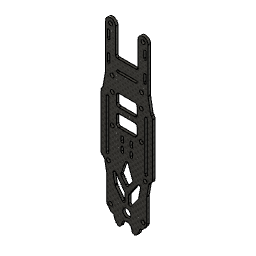
VTX_Mount_Assembly (Autodesk Fusion 360 archive; units mm, degrees)
design "frame_top_2mm"
Autodesk Fusion 360 part; units mm, degrees
(part 1 of 3)
sketch "Sketch1" plane through (0, 0, 0) normal (0, 0, 1) x (1, 0, 0)
  circle A0 centre (15.25, -31.25) radius 1.6
  line L0 (2, 0) -> (13.2991, 0) construction
  line L1 (2, 0) -> (13.2991, 0) construction
  line L2 (9.35, 67.3) -> (9.35, 67.95)
  line L3 (15.95, 56.45) -> (15.95, 62.15)
  circle A1 centre (13.5, 67.95) radius 1.6
  circle A2 centre (13.5, 67.95) radius 4.15
  arc A3 (14.15, 56.45) -> (15.95, 56.45) centre (15.05, 56.45) ccw
  line L4 (14.15, 62.15) -> (14.15, 56.45)
  circle A4 centre (12.2, 31.25) radius 1.6
  line L5 (15.05, 62.15) -> (15.05, 56.45) construction
  arc A5 (15.95, 62.15) -> (14.15, 62.15) centre (15.05, 62.15) ccw
  circle A6 centre (13.45, -61.45) radius 1.6
  line L6 (13.5, 72.1) -> (-2.7063, 72.1) construction
  line L7 (0, 45.6) -> (7.85, 45.6)
  line L8 (9.35, 47.1) -> (9.35, 67.95)
  line L9 (9.35, 67.95) -> (0, 67.95)
  line L10 (0, 67.95) -> (0, 45.6)
  arc A7 (7.85, 45.6) -> (9.35, 47.1) centre (7.85, 47.1) ccw
  circle A8 centre (12, 19.45) radius 1.6
  circle A9 centre (12, -4.55) radius 1.6
  line L11 (17.65, 67.95) -> (17.65, 30.95)
  line L12 (15.95, 39.45) -> (15.95, 45.15)
  arc A10 (15.95, 45.15) -> (14.15, 45.15) centre (15.05, 45.15) ccw
  line L13 (14.15, 45.15) -> (14.15, 39.45)
  line L14 (15.05, 45.15) -> (15.05, 39.45) construction
  arc A11 (14.15, 39.45) -> (15.95, 39.45) centre (15.05, 39.45) ccw
  line L15 (17.65, 30.95) -> (20.0688, 17.2322)
  line L16 (21.35, 19.1304) -> (21.35, -33.1855)
  line L17 (21.35, 17.5398) -> (19.8632, 18.3982)
  circle A12 centre (13.45, -61.45) radius 3.1
  line L18 (16.55, -61.45) -> (16.55, -41.45)
  line L19 (16.55, -41.45) -> (18.6024, -29.8104)
  line L20 (16.55, -41.45) -> (28.3691, -41.45) construction
  line L21 (21.35, -29.1237) -> (18.4258, -30.812)
  line L22 (21.35, -29.1237) -> (17.9734, -29.1237) construction
  arc A13 (11.4643, -67.4123) -> (14.739, -64.2693) centre (10.8143, -63.4576) ccw
  circle A14 centre (0, -71.85) radius 4.25
  line L23 (0, -71.85) -> (0, 0) construction
  line L24 (10.8143, -67.4654) -> (8.5812, -67.4654) construction
  line L25 (6.7155, -73.9955) -> (4.3713, -73.9955) construction
  spline S0 degree 5 poles (10.6535, -68.1682) (10.6286, -68.2734) (10.547, -68.6119) (10.4102, -69.1517) (10.2203, -69.8303) (9.9795, -70.5538) (9.7046, -71.1854) (9.4084, -71.6765) (9.0557, -72.1429) (8.6004, -72.7445) (8.0471, -73.3833) (7.5409, -73.7918) (7.1365, -73.9585) (6.8574, -73.9955) (6.7155, -73.9955) knots 0.056122 0.056122 0.056122 0.056122 0.056122 0.056122 0.1 0.2 0.3 0.4 0.5 0.6 0.7 0.8 0.9 1 1 1 1 1 1
  line L26 (9.6717, -71.2822) -> (8.91, -72.3592)
  arc A15 (4.2449, -71.6427) -> (6.7155, -73.9955) centre (6.7155, -71.5221) ccw
  arc A16 (11.4643, -67.4123) -> (10.6535, -68.1682) centre (11.6265, -68.3991) ccw
  circle A17 centre (0, -61.45) radius 3.35
  line L27 (0, -61.45) -> (13.45, -61.45) construction
  line L28 (-7.55, 35.5) -> (7.55, 35.5)
  arc A18 (7.55, 35.5) -> (7.55, 37.4) centre (7.55, 36.45) ccw
  line L29 (7.55, 37.4) -> (-7.55, 37.4)
  arc A19 (-7.55, 37.4) -> (-7.55, 35.5) centre (-7.55, 36.45) ccw
  line L30 (-8.5, 36.45) -> (8.5, 36.45) construction
  line L31 (0, 36.45) -> (0, 0) construction
  line L32 (-6.6, 21.2) -> (6.6, 21.2)
  line L33 (8.6, 19.2) -> (8.6, 13)
  line L34 (6.6, 11) -> (-6.6, 11)
  line L35 (-8.6, 13) -> (-8.6, 19.2)
  line L36 (-8.6, 21.2) -> (8.6, 11) construction
  line L37 (8.6, 21.2) -> (-8.6, 11) construction
  line L38 (-6.6, 6.6) -> (6.6, 6.6)
  line L39 (8.6, 4.6) -> (8.6, -1.6)
  line L40 (6.6, -3.6) -> (-6.6, -3.6)
  line L41 (-8.6, -1.6) -> (-8.6, 4.6)
  line L42 (-8.6, 6.6) -> (8.6, -3.6) construction
  line L43 (8.6, 6.6) -> (-8.6, -3.6) construction
  arc A20 (-6.6, 6.6) -> (-8.6, 4.6) centre (-6.6, 4.6) ccw
  arc A21 (-8.6, -1.6) -> (-6.6, -3.6) centre (-6.6, -1.6) ccw
  arc A22 (6.6, -3.6) -> (8.6, -1.6) centre (6.6, -1.6) ccw
  arc A23 (8.6, 4.6) -> (6.6, 6.6) centre (6.6, 4.6) ccw
  arc A24 (6.6, 11) -> (8.6, 13) centre (6.6, 13) ccw
  arc A25 (-8.6, 13) -> (-6.6, 11) centre (-6.6, 13) ccw
  arc A26 (-6.6, 21.2) -> (-8.6, 19.2) centre (-6.6, 19.2) ccw
  arc A27 (8.6, 19.2) -> (6.6, 21.2) centre (6.6, 19.2) ccw
  line L44 (2.75, -8.9) -> (2.75, -12)
  arc A28 (2.75, -12) -> (4.75, -12) centre (3.75, -12) ccw
  line L45 (4.75, -12) -> (4.75, -8.9)
  arc A29 (4.75, -8.9) -> (2.75, -8.9) centre (3.75, -8.9) ccw
  line L46 (3.75, -7.9) -> (3.75, -13) construction
  line L47 (2.75, -16.5) -> (2.75, -19.6)
  arc A30 (4.75, -16.5) -> (2.75, -16.5) centre (3.75, -16.5) ccw
  line L48 (3.75, -15.5) -> (3.75, -20.6) construction
  arc A31 (2.75, -19.6) -> (4.75, -19.6) centre (3.75, -19.6) ccw
  line L49 (4.75, -19.6) -> (4.75, -16.5)
  line L50 (14.95, 14.45) -> (14.95, -26.05)
  arc A32 (14.95, -26.05) -> (16.95, -26.05) centre (15.95, -26.05) ccw
  line L51 (16.95, -26.05) -> (16.95, 14.45)
  arc A33 (16.95, 14.45) -> (14.95, 14.45) centre (15.95, 14.45) ccw
  line L52 (15.95, 15.45) -> (15.95, -27.05) construction
  line L53 (0, -22.2) -> (5.1, -36.2121)
  line L54 (5.1, -36.2121) -> (0, -43.2)
  line L55 (1.45, -54.0214) -> (1.45, -48.0614)
  line L56 (1.6739, -47.3475) -> (10.5932, -34.5275)
  line L57 (9.8726, -46.033) -> (12.1558, -33.9583)
  line L58 (9.6573, -46.5332) -> (3.7129, -54.7538)
  arc A34 (11.3939, -37.9877) -> (8.9108, -36.9456) centre (10.041, -37.7319) ccw
  arc A35 (9.6573, -46.5332) -> (9.8726, -46.033) centre (8.6443, -45.8007) ccw
  arc A36 (1.6739, -47.3475) -> (1.45, -48.0614) centre (2.7, -48.0614) ccw
  arc A37 (1.45, -54.0214) -> (3.7129, -54.7538) centre (2.7, -54.0214) ccw
  arc A38 (-8.6, 13) -> (-6.6, 11) centre (-6.6, 13) ccw
  arc A39 (-15.95, 39.45) -> (-14.15, 39.45) centre (-15.05, 39.45) ccw
  line L59 (0, 67.95) -> (0, 45.6)
  line L60 (0, 36.45) -> (0, 0) construction
  circle A40 centre (-13.45, -61.45) radius 1.6
  line L61 (-3.75, -15.5) -> (-3.75, -20.6) construction
  arc A41 (-1.45, -48.0614) -> (-1.6739, -47.3475) centre (-2.7, -48.0614) ccw
  arc A42 (-4.75, -12) -> (-2.75, -12) centre (-3.75, -12) ccw
  line L62 (-21.35, -29.1237) -> (-17.9734, -29.1237) construction
  line L63 (-16.55, -41.45) -> (-18.6024, -29.8104)
  line L64 (-4.75, -19.6) -> (-4.75, -16.5)
  circle A43 centre (-15.25, -31.25) radius 1.6
  line L65 (-14.15, 45.15) -> (-14.15, 39.45)
  arc A44 (-8.9108, -36.9456) -> (-11.3939, -37.9877) centre (-10.041, -37.7319) ccw
  arc A45 (-14.739, -64.2693) -> (-11.4643, -67.4123) centre (-10.8143, -63.4576) ccw
  line L66 (-21.35, 19.1304) -> (-21.35, -33.1855)
  line L67 (-14.95, 14.45) -> (-14.95, -26.05)
  line L68 (-16.95, -26.05) -> (-16.95, 14.45)
  circle A46 centre (-13.45, -61.45) radius 3.1
  line L69 (0, -61.45) -> (-13.45, -61.45) construction
  line L70 (-9.6573, -46.5332) -> (-3.7129, -54.7538)
  line L71 (-15.95, 56.45) -> (-15.95, 62.15)
  line L72 (-9.35, 67.95) -> (0, 67.95)
  line L73 (0, 45.6) -> (-7.85, 45.6)
  line L74 (-8.6, 19.2) -> (-8.6, 13)
  line L75 (-21.35, 17.5398) -> (-19.8632, 18.3982)
  line L76 (-14.15, 62.15) -> (-14.15, 56.45)
  arc A47 (-14.15, 62.15) -> (-15.95, 62.15) centre (-15.05, 62.15) ccw
  circle A48 centre (-13.5, 67.95) radius 4.15
  line L77 (-15.05, 62.15) -> (-15.05, 56.45) construction
  line L78 (-8.6, 4.6) -> (-8.6, -1.6)
  line L79 (-15.95, 39.45) -> (-15.95, 45.15)
  line L80 (-9.35, 47.1) -> (-9.35, 67.95)
  line L81 (-9.35, 67.3) -> (-9.35, 67.95)
  arc A49 (-6.6, 6.6) -> (-8.6, 4.6) centre (-6.6, 4.6) ccw
  arc A50 (-7.55, 37.4) -> (-7.55, 35.5) centre (-7.55, 36.45) ccw
  arc A51 (-15.95, 56.45) -> (-14.15, 56.45) centre (-15.05, 56.45) ccw
  line L82 (-1.45, -54.0214) -> (-1.45, -48.0614)
  line L83 (-2.75, -16.5) -> (-2.75, -19.6)
  line L84 (-2.75, -8.9) -> (-2.75, -12)
  line L85 (-4.75, -12) -> (-4.75, -8.9)
  arc A52 (-2.75, -8.9) -> (-4.75, -8.9) centre (-3.75, -8.9) ccw
  line L86 (-3.75, -7.9) -> (-3.75, -13) construction
  arc A53 (-2.75, -16.5) -> (-4.75, -16.5) centre (-3.75, -16.5) ccw
  arc A54 (-4.75, -19.6) -> (-2.75, -19.6) centre (-3.75, -19.6) ccw
  circle A55 centre (-12.2, 31.25) radius 1.6
  circle A56 centre (-13.5, 67.95) radius 1.6
  line L87 (-15.95, 15.45) -> (-15.95, -27.05) construction
  line L88 (-17.65, 30.95) -> (-20.0688, 17.2322)
  line L89 (-15.05, 45.15) -> (-15.05, 39.45) construction
  line L90 (-17.65, 67.95) -> (-17.65, 30.95)
  arc A57 (-6.6, 21.2) -> (-8.6, 19.2) centre (-6.6, 19.2) ccw
  circle A58 centre (-12, 19.45) radius 1.6
  arc A59 (-14.15, 45.15) -> (-15.95, 45.15) centre (-15.05, 45.15) ccw
  arc A60 (-9.35, 47.1) -> (-7.85, 45.6) centre (-7.85, 47.1) ccw
  arc A61 (-14.95, 14.45) -> (-16.95, 14.45) centre (-15.95, 14.45) ccw
  circle A62 centre (-12, -4.55) radius 1.6
  line L91 (-2, 0) -> (-13.2991, 0) construction
  line L92 (-2, 0) -> (-13.2991, 0) construction
  line L93 (-21.35, -29.1237) -> (-18.4258, -30.812)
  line L94 (-1.6739, -47.3475) -> (-10.5932, -34.5275)
  arc A63 (-8.6, -1.6) -> (-6.6, -3.6) centre (-6.6, -1.6) ccw
  line L95 (-9.8726, -46.033) -> (-12.1558, -33.9583)
  line L96 (0, -22.2) -> (-5.1, -36.2121)
  arc A64 (-16.95, -26.05) -> (-14.95, -26.05) centre (-15.95, -26.05) ccw
  arc A65 (-9.8726, -46.033) -> (-9.6573, -46.5332) centre (-8.6443, -45.8007) ccw
  line L97 (-16.55, -61.45) -> (-16.55, -41.45)
  line L98 (-5.1, -36.2121) -> (0, -43.2)
  arc A66 (-3.7129, -54.7538) -> (-1.45, -54.0214) centre (-2.7, -54.0214) ccw
  line L99 (-6.7155, -73.9955) -> (-4.3713, -73.9955) construction
  arc A67 (-6.7155, -73.9955) -> (-4.2449, -71.6427) centre (-6.7155, -71.5221) ccw
  spline S1 degree 5 poles (-10.6535, -68.1682) (-10.6286, -68.2734) (-10.547, -68.6119) (-10.4102, -69.1517) (-10.2203, -69.8303) (-9.9795, -70.5538) (-9.7046, -71.1854) (-9.4084, -71.6765) (-9.0557, -72.1429) (-8.6004, -72.7445) (-8.0471, -73.3833) (-7.5409, -73.7918) (-7.1365, -73.9585) (-6.8574, -73.9955) (-6.7155, -73.9955) knots 0.056122 0.056122 0.056122 0.056122 0.056122 0.056122 0.1 0.2 0.3 0.4 0.5 0.6 0.7 0.8 0.9 1 1 1 1 1 1
  line L100 (10.9009, -67.1253) -> (10.4061, -69.2111)
  line L101 (7.7873, -73.9955) -> (5.6436, -73.9955)
  line L102 (-10.9009, -67.1253) -> (-10.4061, -69.2111)
  line L103 (-9.6717, -71.2822) -> (-8.91, -72.3592)
  line L104 (-7.7873, -73.9955) -> (-5.6436, -73.9955)
  arc A68 (-10.6535, -68.1682) -> (-11.4643, -67.4123) centre (-11.6265, -68.3991) ccw
  point P0 (9.2908, -71.8207)
  point P1 (0, 36.45)
  point P2 (0, 16.1)
  point P3 (0, 1.5)
  point P4 (-8.6, 6.6)
  point P5 (0, 1.5)
  point P6 (0, 16.1)
  point P7 (0, -61.45)
  point P8 (-8.5, 36.45)
  point P9 (-8.6, -3.6)
  point P10 (-8.6, 11)
  point P11 (-8.6, 21.2)
  point P12 (-13.5, 72.1)
  point P13 (0, 36.45)
  point P14 (0, -71.85)
  point P15 (-9.2908, -71.8207)
  point P16 (0, -71.85)
  dimension "d29" = 30.2
  dimension "d49" = 1.8
  dimension "d50" = 5.7
  dimension "d52" = 5.8
  dimension "d65" = 3.2
  dimension "d66" = 26.5
  dimension "d67" = 8.3
  dimension "d68" = 31.25
  dimension "d69" = 15.25
  dimension "d71" = 31.25
  dimension "d72" = 12.2
  dimension "d73" = 36.7
  dimension "d74" = 13.5
  dimension "d75" = 1.5
  dimension "d76" = 11.8
  dimension "d77" = 24
  dimension "d78" = 12
  dimension "d79" = 12
  dimension "d80" = 13.45
  dimension "d81" = 37
  dimension "d82" = 1.7
  dimension "d83" = 1.8
  dimension "d84" = 5.7
  dimension "d85" = 1.7
  dimension "d86" = 11.3
  dimension "d87" = 21.35
  dimension "d88" = 120
  dimension "d89" = 170
  dimension "d90" = 6.2
  dimension "d91" = 20
  dimension "d92" = 80
  dimension "d93" = 30
  dimension "d94" = 8.5
  dimension "d96" = 1
  dimension "d97" = 6.7
  dimension "d98" = 17
  dimension "d99" = 1.9
  dimension "d100" = 8.2
  dimension "d101" = 17.2
  dimension "d102" = 10.2
  dimension "d103" = 14.3
  dimension "d104" = 17.2
  dimension "d105" = 10.2
  dimension "d106" = 4.4
  dimension "d107" = 2
  dimension "d108" = 2
  dimension "d109" = 5.1
  dimension "d110" = 4.3
  dimension "d111" = 2.75
  dimension "d114" = 0
  dimension "d115" = -7.6
  dimension "d116" = 2
  dimension "d117" = 42.5
  dimension "d118" = 4.4
  dimension "d119" = 4.2
  dimension "d120" = 10.4
  dimension "d121" = 5.1
  dimension "d122" = 22.2
  dimension "d123" = 21
  dimension "d124" = 20
  dimension "d125" = 1.45
  dimension "d126" = 1.25
  constraint concentric A1 A2
  constraint coincident L2.end A2
  constraint vertical L2
  constraint tangent L2 A2
  constraint tangent A3 L4
  constraint tangent L3 A3
  constraint parallel L3 L4
  constraint tangent L3 A5
  constraint tangent L4 A5
  constraint coincident A2 L6.start
  constraint horizontal L6
  constraint tangent A2 L6
  constraint horizontal L7
  constraint vertical L8
  constraint horizontal L9
  constraint vertical L10
  constraint equal A0 A6
  constraint equal A0 A4
  constraint equal A1 A4
  constraint coincident L23.end L10
  constraint tangent L7 A7
  constraint tangent L8 A7
  constraint equal A8 A9
  constraint equal A1 A8
  constraint coincident A2 L11.start
  constraint vertical L11
  constraint tangent A2 L11
  constraint tangent L13 A11
  constraint tangent L12 A11
  constraint parallel L12 L13
  constraint tangent L12 A10
  constraint tangent A10 L13
  constraint vertical L16
  constraint coincident L16 L17.start
  constraint coincident L15 L17.end
  constraint concentric A6 A12
  constraint coincident A12 L18.start
  constraint tangent A12 L18
  constraint vertical L18
  constraint horizontal L20
  constraint horizontal L22
  constraint coincident L16 L21.start
  constraint coincident L19 L21.end
  constraint coincident A12 A13.end
  constraint coincident P16 P14
  constraint coincident L23.end L31.end
  constraint vertical L23
  constraint horizontal L24
  constraint tangent A13 L24
  constraint horizontal L25
  constraint midpoint P0 L26
  constraint tangent L25 A15
  constraint coincident A14 A15.start
  constraint tangent A14 A15
  constraint coincident L24.start A13
  constraint tangent A13 A16
  constraint tangent S0 A16
  constraint coincident L23 P7
  constraint coincident P7 A17.centre
  constraint coincident A6.centre A12.centre
  constraint horizontal L27
  constraint tangent L28 A18
  constraint tangent A18 L29
  constraint parallel L28 L29
  constraint tangent L29 A19
  constraint tangent L28 A19
  constraint midpoint A19 P8
  constraint midpoint A18 L30.end
  constraint horizontal L30
  constraint midpoint L30 P13
  constraint coincident P13 P1
  constraint vertical L31
  constraint horizontal L32
  constraint perpendicular L32 L33
  constraint parallel L32 L34
  constraint parallel L33 L35
  constraint coincident L36 P6
  constraint coincident L37 P6
  constraint coincident L31 P6
  constraint horizontal L38
  constraint perpendicular L38 L39
  constraint parallel L38 L40
  constraint parallel L39 L41
  constraint coincident L42 P5
  constraint coincident L43 P5
  constraint coincident L31 P5
  constraint coincident P4 L38
  constraint coincident P4 L41
  constraint tangent L38 A20
  constraint tangent L41 A20
  constraint coincident P9 L41
  constraint coincident P9 L40
  constraint tangent L41 A21
  constraint tangent L40 A21
  constraint equal A20 A21
  constraint coincident L42.end L40
  constraint coincident L42.end L39
  constraint tangent L40 A22
  constraint tangent L39 A22
  constraint equal A20 A22
  constraint coincident L43.start L39
  constraint coincident L43.start L38
  constraint tangent L39 A23
  constraint tangent L38 A23
  constraint equal A20 A23
  constraint coincident L36.end L34
  constraint coincident L36.end L33
  constraint tangent L34 A24
  constraint tangent L33 A24
  constraint equal A20 A24
  constraint coincident P10 L34
  constraint coincident P10 L35
  constraint tangent L34 A25
  constraint tangent L35 A25
  constraint equal A20 A25
  constraint coincident P11 L35
  constraint coincident P11 L32
  constraint tangent L35 A26
  constraint tangent L32 A26
  constraint equal A20 A26
  constraint coincident L37.start L32
  constraint coincident L37.start L33
  constraint tangent L32 A27
  constraint tangent L33 A27
  constraint equal A20 A27
  constraint tangent L44 A28
  constraint tangent A28 L45
  constraint parallel L44 L45
  constraint tangent L45 A29
  constraint tangent L44 A29
  constraint midpoint A29 L46.start
  constraint midpoint A28 L46.end
  constraint vertical L46
  constraint tangent L50 A32
  constraint tangent A32 L51
  constraint parallel L50 L51
  constraint tangent L51 A33
  constraint tangent L50 A33
  constraint midpoint A33 L52.start
  constraint midpoint A32 L52.end
  constraint vertical L52
  constraint coincident L23 L53.start
  constraint coincident L23 L54.end
  constraint vertical L55
  constraint tangent L57 A34
  constraint coincident L57 A34.start
  constraint coincident L56 A34.end
  constraint tangent L56 A34
  constraint tangent L57 A35
  constraint tangent L58 A35
  constraint tangent L56 A36
  constraint tangent L55 A36
  constraint equal A35 A36
  constraint tangent L58 A37
  constraint tangent L55 A37
  constraint equal A35 A37
  constraint midpoint S0.start L100
  constraint midpoint L25.start L101
  constraint symmetric L31.end L23 L60.end
  constraint symmetric L4.start L23 L76.start
  constraint symmetric A3.start L23 L76.end
  constraint symmetric L3.start L23 L71.start
  constraint symmetric L3.end L23 L71.end
  constraint symmetric L0.start L23 L91.start
  constraint symmetric L0.end L23 L91.end
  constraint symmetric L2.start L23 L81.start
  constraint symmetric L2.end L23 L72.start
  constraint symmetric A0 L23 A43
  constraint symmetric A1 L23 A56
  constraint symmetric A2 L23 A48
  constraint symmetric A3 L23 A51
  constraint symmetric A4 L23 A55
  constraint symmetric A5 L23 A47
  constraint symmetric A6 L23 A40
  constraint symmetric L6.start L23 P12
  constraint symmetric L7.start L23 L10.end
  constraint symmetric L9.end L23 L10.start
  constraint symmetric L7.end L23 L73.end
  constraint symmetric L8.start L23 L80.start
  constraint symmetric A7 L23 A60
  constraint symmetric A8 L23 A58
  constraint symmetric A9 L23 A62
  constraint symmetric L11.start L23 L90.start
  constraint symmetric L11.end L23 L88.start
  constraint symmetric L12.end L23 L79.end
  constraint symmetric L12.start L23 A39.start
  constraint symmetric L13.end L23 A39.end
  constraint symmetric A10.end L23 L65.start
  constraint symmetric A10 L23 A59
  constraint symmetric A11 L23 A39
  constraint symmetric L15.end L23 L88.end
  constraint symmetric L16.start L23 L66.start
  constraint symmetric L16.end L23 L66.end
  constraint symmetric L17.start L23 L75.start
  constraint symmetric L17.end L23 L75.end
  constraint symmetric A12 L23 A46
  constraint symmetric L18.start L23 L97.start
  constraint symmetric L18.end L23 L63.start
  constraint symmetric L19.end L23 L63.end
  constraint symmetric L21.start L23 L62.start
  constraint symmetric L21.end L23 L93.end
  constraint symmetric L22.end L23 L62.end
  constraint symmetric A13.end L23 A45.start
  constraint symmetric A13 L23 A45
  constraint symmetric P16 L23 P14
  constraint symmetric L23 L25.start L99.start
  constraint symmetric L23 L25.end L99.end
  constraint symmetric L23 P0 P15
  constraint symmetric L23 L26.start L103.start
  constraint symmetric L23 L26.end L103.end
  constraint symmetric L23 A15.start A67.end
  constraint symmetric L23 A15 A67
  constraint symmetric L23 S0.start S1.start
  constraint symmetric L23 A13.start A45.end
  constraint symmetric L23 P7 A17.centre
  constraint symmetric L23 A6.centre A40.centre
  constraint symmetric L23 L28.end L28.start
  constraint symmetric L23 A18.end L29.end
  constraint symmetric L23 A18 A50
  constraint symmetric L23 L30.end P8
  constraint symmetric L23 P13 P1
  constraint symmetric L23 L37.start P11
  constraint symmetric L23 L36.end P10
  constraint symmetric L23 P6 P2
  constraint symmetric L23 L43.start P4
  constraint symmetric L23 L42.end P9
  constraint symmetric L23 P5 P3
  constraint symmetric L23 L40.start L40.end
  constraint symmetric L23 L39.end L41.start
  constraint symmetric L23 A22 A63
  constraint symmetric L23 L39.start L41.end
  constraint symmetric L23 L38.end L38.start
  constraint symmetric L23 A23 A49
  constraint symmetric L23 L34.start L34.end
  constraint symmetric L23 L33.end L35.start
  constraint symmetric L23 A24 A38
  constraint symmetric L23 L32.end L32.start
  constraint symmetric L23 L33.start L35.end
  constraint symmetric L23 A27 A57
  constraint symmetric L23 L44.start L84.start
  constraint symmetric L23 L44.end A42.end
  constraint symmetric L23 A28.end A42.start
  constraint symmetric L23 L45.end L85.end
  constraint symmetric L23 A28 A42
  constraint symmetric L23 A29 A52
  constraint symmetric L23 L46.start L86.start
  constraint symmetric L23 L46.end L86.end
  constraint symmetric L23 A31.end L64.start
  constraint symmetric L23 L47.start L83.start
  constraint symmetric L23 L47.end L83.end
  constraint symmetric L23 L48.end L61.end
  constraint symmetric L23 A30.start L64.end
  constraint symmetric L23 A30 A53
  constraint symmetric L23 L48.start L61.start
  constraint symmetric L23 A31 A54
  constraint symmetric L23 L50.start L67.start
  constraint symmetric L23 L50.end L67.end
  constraint symmetric L23 A32.end L68.start
  constraint symmetric L23 L51.end L68.end
  constraint symmetric L23 A32 A64
  constraint symmetric L23 A33 A61
  constraint symmetric L23 L52.start L87.start
  constraint symmetric L23 L52.end L87.end
  constraint symmetric L23 L53.start L96.start
  constraint symmetric L23 L53.end L96.end
  constraint symmetric L23 L54.end L98.end
  constraint symmetric L23 L56.end L94.end
  constraint symmetric L23 L57.end L95.end
  constraint symmetric L23 A34.end A44.start
  constraint symmetric L23 A34.start A44.end
  constraint symmetric L23 A34 A44
  constraint symmetric L23 L57.start L95.start
  constraint symmetric L23 L58.start L70.start
  constraint symmetric L23 A35 A65
  constraint symmetric L23 L56.start A41.end
  constraint symmetric L23 L55.end A41.start
  constraint symmetric L23 A36 A41
  constraint symmetric L23 L58.end L70.end
  constraint symmetric L23 L55.start L82.start
  constraint symmetric L23 A37 A66
  constraint symmetric L23 L100.start L102.start
  constraint symmetric L23 L100.end L102.end
  constraint symmetric L23 L101.start L104.start
  constraint symmetric L23 L101.end L104.end
  constraint tangent A45 A68
  measures "d29" vertical distance of A0.centre A6.centre
  measures "d49" distance of L3 L4
  measures "d50" distance of L5.start A3.centre
  measures "d52" vertical distance of L5.start A1.centre
  measures "d65" diameter of A1
  measures "d66" distance of L6 L7
  measures "d67" diameter of A2
  measures "d68" vertical distance of L23.end A0.centre
  measures "d69" horizontal distance of L23.end A0.centre
  measures "d71" vertical distance of L23.end A4.centre
  measures "d72" horizontal distance of L23.end A4.centre
  measures "d73" vertical distance of A1.centre A4.centre
  measures "d74" horizontal distance of L23.end A1.centre
  measures "d75" radius of A7
  measures "d76" vertical distance of A4.centre A8.centre
  measures "d77" distance of A8.centre A9.centre
  measures "d78" horizontal distance of L23.end A8.centre
  measures "d79" horizontal distance of L23.end A9.centre
  measures "d80" horizontal distance of L23.end A6.centre
  measures "d81" distance of L11.start L11.end
  measures "d82" distance of L3 L11
  measures "d83" distance of L12 L13
  measures "d84" distance of L14.end A10.centre
  measures "d85" distance of L11 L12
  measures "d86" distance of A3.centre A10.centre
  measures "d87" distance of L23.end L16
  measures "d88" angle of L16 L17
  measures "d89" angle of L11 L15
  measures "d90" diameter of A12
  measures "d91" distance of L18.start L18.end
  measures "d92" angle of L19 L20
  measures "d93" angle of L21 L22
  measures "d94" diameter of A14
  measures "d96" radius of A16
  measures "d97" diameter of A17
  measures "d98" distance of P8 L30.end
  measures "d99" distance of L28 L29
  measures "d100" distance of L7 L29
  measures "d101" distance of L36.end P10
  measures "d102" distance of L37.start L36.end
  measures "d103" distance of L28 L32
  measures "d104" distance of L42.end P9
  measures "d105" distance of L43.start L42.end
  measures "d106" distance of L34 L38
  measures "d107" radius of A20
  measures "d108" diameter of A28
  measures "d109" distance of L46.start L46.end
  measures "d110" distance of L40 L46.start
  measures "d111" distance of L23 L44
  measures "d116" diameter of A32
  measures "d117" distance of L52.start L52.end
  measures "d118" distance of L16 L51
  measures "d119" vertical distance of A0.centre L52.end
  measures "d120" distance of P16 P7
  measures "d121" distance of L23 L53.end
  measures "d122" distance of L23.end L53.start
  measures "d123" distance of L53.start L54.end
  measures "d124" angle of L23 L53
  measures "d125" distance of L23 L55
  measures "d126" radius of A35
extrude "Extrude1" add sketch "Sketch1" along normal blind 2 contours L2 A2 L7 L8 A7 L11 L15 L16 L17 A12 L18 L19 L21 A13 A14 S0 A15 A16 L63 A45 L66 A46 L73 L75 A48 L80 L81 L88 L90 A60 L93 L97 A67 S1 A68 | A2 | A48 | A12 | A46
fillet "Fillet1" radius 1.25 4 edges at (0, -22.2, 1) (0, -43.2, 1) (-5.1, -36.2121, 1) (5.1, -36.2121, 1)
fillet "Fillet2" radius 2 2 edges at (14.739, -64.2693, 1) (-14.739, -64.2693, 1)
fillet "Fillet3" radius 3 12 edges at (18.4258, -30.812, 1) (21.35, -29.1237, 1) (-18.4258, -30.812, 1) (-21.35, -29.1237, 1) (-21.35, 17.5398, 1) (-19.8632, 18.3982, 1) (21.35, 17.5398, 1) (19.8632, 18.3982, 1) (17.65, 30.95, 1) (-17.65, 30.95, 1) (-16.55, -41.45, 1) (16.55, -41.45, 1)
equation "d78 = ( 24 / 2 ) * 1 mm"
equation "d79 = d78"
equation "d80 = ( 26.9 / 2 ) * 1 mm"
equation "d86 = 9.5 mm + d49"
equation "d87 = ( 42.7 / 2 ) * 1 mm"
equation "d111 = ( 5.5 / 2 ) * 1 mm"
equation "d119 = 2.6 mm + ( d65 / 2 )"
equation "d120 = d97 / 2 + d94 / 2 + 2.8 mm"
equation "d125 = ( 2.9 / 2 ) * 1 mm"

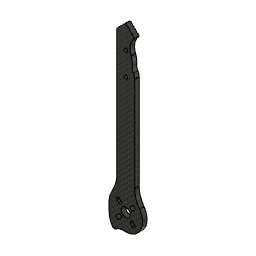
design "frame_arm_4mm"
Autodesk Fusion 360 part; units mm, degrees
sketch "Sketch3" plane through (0, 0, 0) normal (0, 0, 1) x (1, 0, 0)
  circle A0 centre (0.0083, -64.5282) radius 4.05
  circle A1 centre (0.0083, -64.5282) radius 8.75 construction
  line L0 (0.0083, -64.5282) -> (6.1955, -58.341) construction
  line L1 (0.0083, -64.5282) -> (8.7583, -64.5282) construction
  line L2 (6.4784, -60.1795) -> (8.034, -58.6238)
  arc A2 (8.034, -58.6238) -> (5.9127, -56.5025) centre (6.9733, -57.5632) ccw
  line L3 (5.9127, -56.5025) -> (4.357, -58.0581)
  arc A3 (4.357, -58.0581) -> (6.4784, -60.1795) centre (5.4177, -59.1188) ccw
  line L4 (4.357, -60.1795) -> (8.034, -56.5025) construction
  line L5 (4.357, -60.1795) -> (7.9558, -60.1795) construction
  line L6 (-4.3404, -58.0581) -> (-5.896, -56.5025)
  line L7 (-8.0173, -58.6238) -> (-6.4617, -60.1795)
  arc A4 (-6.4617, -60.1795) -> (-4.3404, -58.0581) centre (-5.401, -59.1188) ccw
  line L8 (-4.3404, -60.1795) -> (-8.0173, -56.5025) construction
  arc A5 (-5.896, -56.5025) -> (-8.0173, -58.6238) centre (-6.9567, -57.5632) ccw
  line L9 (-6.4617, -68.8769) -> (-8.0173, -70.4325)
  line L10 (-5.896, -72.5538) -> (-4.3404, -70.9982)
  arc A6 (-4.3404, -70.9982) -> (-6.4617, -68.8769) centre (-5.401, -69.9375) ccw
  line L11 (-4.3404, -68.8769) -> (-8.0173, -72.5538) construction
  arc A7 (-8.0173, -70.4325) -> (-5.896, -72.5538) centre (-6.9567, -71.4932) ccw
  line L12 (4.357, -70.9982) -> (5.9127, -72.5538)
  line L13 (8.034, -70.4325) -> (6.4784, -68.8769)
  arc A8 (6.4784, -68.8769) -> (4.357, -70.9982) centre (5.4177, -69.9375) ccw
  line L14 (4.357, -68.8769) -> (8.034, -72.5538) construction
  arc A9 (5.9127, -72.5538) -> (8.034, -70.4325) centre (6.9733, -71.4932) ccw
  circle A10 centre (0.0083, -64.5282) radius 15.1
  line L15 (-8.8515, -81.7805) -> (-9.2245, -82.0856)
  line L16 (-11.4526, -81.7512) -> (-11.2758, -81.9426)
  arc A11 (-1.4818, -79.5545) -> (-8.8515, -81.7805) centre (-2.4756, -89.5764) ccw
  line L17 (0.0083, -64.5282) -> (-15.0917, -64.5282) construction
  spline S0 degree 5 poles (-11.4526, -81.7512) (-11.5434, -81.653) (-11.7181, -81.4571) (-11.959, -81.1655) (-12.2453, -80.7768) (-12.5785, -80.2658) (-12.9207, -79.695) (-13.2839, -79.026) (-13.6569, -78.2216) (-14.017, -77.2506) (-14.3381, -76.0931) (-14.6006, -74.7468) (-14.7984, -73.2325) (-14.9351, -71.5854) (-15.0206, -69.8489) (-15.0676, -68.0675) (-15.0846, -66.6385) (-15.0904, -65.5777) (-15.0917, -64.8769) (-15.0917, -64.5282) knots 0 0 0 0 0 0 0.066667 0.133333 0.2 0.266667 0.333333 0.4 0.466667 0.533333 0.6 0.666667 0.733333 0.8 0.866667 0.933333 1 1 1 1 1 1
  arc A12 (-11.2758, -81.9426) -> (-9.2245, -82.0856) centre (-10.1742, -80.9245) ccw
  line L18 (0, 0) -> (-8.1, 0) construction
  line L19 (-8.1, 0) -> (-8.1, 74.424)
  line L20 (-8.1, 0) -> (-8.1, -40.576)
  spline S1 degree 5 poles (-15.0917, -64.5282) (-15.0917, -64.2457) (-15.0821, -63.684) (-15.0388, -62.8507) (-14.9249, -61.7598) (-14.6973, -60.4356) (-14.3963, -59.1591) (-14.0349, -57.9381) (-13.626, -56.7786) (-13.1797, -55.6822) (-12.7048, -54.6455) (-12.2091, -53.6579) (-11.7011, -52.7014) (-11.1912, -51.7478) (-10.6919, -50.7589) (-10.216, -49.6979) (-9.7711, -48.5441) (-9.3608, -47.2978) (-8.9724, -46.0117) (-8.6188, -44.7062) (-8.3284, -43.3781) (-8.1734, -42.2856) (-8.1133, -41.4415) (-8.1, -40.8665) (-8.1, -40.576) knots 0 0 0 0 0 0 0.05 0.1 0.15 0.2 0.25 0.3 0.35 0.4 0.45 0.5 0.55 0.6 0.65 0.7 0.75 0.8 0.85 0.9 0.95 1 1 1 1 1 1
  line L21 (-10.3594, -50.3117) -> (-8.6813, -45.2176)
  line L22 (-8.1, 74.424) -> (-0.039, 82.4851)
  line L23 (-8.1, 74.424) -> (3.05, 74.424) construction
  line L24 (-0.039, 82.4851) -> (8.022, 74.424)
  line L25 (-0.039, 82.4851) -> (11.1696, 82.4851) construction
  line L26 (8.022, 74.424) -> (18.0806, 64.3654) construction
  arc A13 (8.022, 74.424) -> (4.8004, 59.2677) centre (18.0806, 64.3654) ccw
  line L27 (18.0806, 64.3654) -> (8.022, 74.424) construction
  line L28 (18.0806, 64.3654) -> (4.8004, 59.2677) construction
  spline S2 degree 5 poles (4.8004, 59.2677) (4.8494, 59.1404) (4.9423, 58.8866) (5.0666, 58.5087) (5.2043, 58.0107) (5.3432, 57.4017) (5.4642, 56.809) (5.5795, 56.2321) (5.6934, 55.6644) (5.7974, 55.0914) (5.8765, 54.4957) (5.916, 53.8616) (5.9073, 53.1806) (5.8552, 52.4567) (5.782, 51.71) (5.7191, 50.9686) (5.6999, 50.2615) (5.7511, 49.6111) (5.8867, 49.0267) (6.0971, 48.4946) (6.3562, 47.9853) (6.5772, 47.5687) (6.7385, 47.238) (6.8424, 47.0077) (6.8934, 46.89) knots 0 0 0 0 0 0 0.05 0.1 0.15 0.2 0.25 0.3 0.35 0.4 0.45 0.5 0.55 0.6 0.65 0.7 0.75 0.8 0.85 0.9 0.95 1 1 1 1 1 1
  line L29 (4.1339, 60.9997) -> (5.467, 57.5357) construction
  line L30 (6.1548, 48.5926) -> (7.632, 45.1875) construction
  circle A14 centre (-0.1012, 42.8053) radius 8.1 construction
  circle A15 centre (0, 61.4851) radius 1.6
  circle A16 centre (0, 40.6251) radius 1.6
  circle A17 centre (-0.1012, 42.8053) radius 8.1
  line L31 (0, 0) -> (0, 40.6251)
  line L32 (-0.1012, 42.8053) -> (7.9988, 42.8053) construction
  line L33 (7.9988, 42.8053) -> (7.9988, -42.1947)
  arc A18 (7.9988, -42.1947) -> (12.3295, -55.799) centre (31.5321, -42.1947) ccw
  point P0 (6.1955, -58.341)
  point P1 (-6.1789, -58.341)
  point P2 (-6.1789, -58.341)
  point P3 (-6.1789, -70.7154)
  point P4 (-6.1789, -70.7154)
  point P5 (6.1955, -70.7154)
  point P6 (6.1955, -70.7154)
  point P7 (-12.7288, -80.0085)
  point P8 (-14.2896, -76.1896)
  point P9 (-13.921, -57.6445)
  point P10 (-11.7496, -52.7944)
  point P11 (-9.5204, -47.7647)
  point P12 (5.9008, 53.2841)
  point P13 (5.5742, 56.2588)
  point P14 (5.7979, 49.475)
  dimension "d1" = 8.1
  dimension "d2" = 17.5
  dimension "d3" = 45
  dimension "d4" = 5.2
  dimension "d5" = 45
  dimension "d6" = 3
  dimension "d8" = 360
  dimension "d9" = 30.2
  dimension "d10" = 1.5
  dimension "d11" = 8.1
  dimension "d12" = 115
  dimension "d13" = 45
  dimension "d14" = 11.4
  dimension "d15" = 45
  dimension "d16" = 11.4
  dimension "d17" = 14.225
  dimension "d18" = 66
  dimension "d19" = 3.2
  dimension "d20" = 21
  dimension "d21" = 3.2
  dimension "d22" = 20.86
  dimension "d23" = 16.2
  dimension "d24" = 85
  constraint concentric A0 A1
  constraint horizontal L1
  constraint coincident A0.centre A1.centre
  constraint coincident A1 P0
  constraint tangent L2 A2
  constraint tangent A2 L3
  constraint parallel L2 L3
  constraint tangent L3 A3
  constraint tangent L2 A3
  constraint midpoint A3 L4.start
  constraint midpoint A2 L4.end
  constraint coincident L0 L4.start
  constraint parallel L0 L4
  constraint midpoint L4 P0
  constraint coincident P0 L0.end
  constraint concentric A1 A10
  constraint tangent L15 A11
  constraint coincident A10 A11.start
  constraint tangent A10 A11
  constraint coincident A10 L17.end
  constraint parallel L1 L17
  constraint tangent A10 S0
  constraint tangent L15 A12
  constraint tangent L16 A12
  constraint coincident L18.start L31.start
  constraint horizontal L18
  constraint perpendicular L18 L19
  constraint perpendicular L18 L20
  constraint tangent A10 S1
  constraint midpoint P11 L21
  constraint horizontal L23
  constraint horizontal L25
  constraint perpendicular L22 L26
  constraint coincident L26.end A13.centre
  constraint coincident S2.end A14
  constraint midpoint A13.end L29
  constraint midpoint S2.end L30
  constraint coincident A16.centre L31.end
  constraint perpendicular L18 L31
  constraint coincident A14.centre A17.centre
  constraint horizontal L32
  constraint coincident A17 L32.end
  constraint coincident A14 L32.end
  constraint perpendicular L32 L33
  constraint tangent A10 A18
  constraint coincident A10 A18.end
  constraint tangent L33 A18
  measures "d1" diameter of A0
  measures "d2" diameter of A1
  measures "d3" angle of L0 L1
  measures "d4" distance of L4.start L4.end
  measures "d5" angle of L4 L5
  measures "d6" diameter of A2
  measures "d9" diameter of A10
  measures "d10" radius of A12
  measures "d11" distance of L18.start L18.end
  measures "d12" distance of L19.end L20.end
  measures "d13" angle of L22 L23
  measures "d14" distance of L19.end L22.end
  measures "d15" angle of L24 L25
  measures "d16" distance of L22.end L24.end
  measures "d17" distance of L24.end L26.end
  measures "d18" angle of L27 L28
  measures "d19" diameter of A15
  measures "d20" vertical distance of L22.end A15.centre
  measures "d21" diameter of A16
  measures "d22" distance of A15.centre A16.centre
  measures "d23" diameter of A14
  measures "d24" distance of L32.end L33.end
extrude "Extrude1" add sketch "Sketch3" along normal blind 4 contours A10 L19 L20 S1 A17 L33 A18 | A10 L15 L16 A11 S0 A12 | L19 A17 | L19 L22 L24 A13 S2 A17 picked at (-5.8704, 42.33)
equation "d2 = d1 + ( ( 2.1 * 2 ) * 1 mm ) + ( 5.2 mm )"
equation "d11 = ( 16.2 / 2 ) * 1 mm"

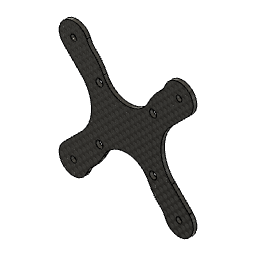
design "frame_bot_2mm"
Autodesk Fusion 360 part; units mm, degrees
sketch "Sketch1" plane through (0, 0, 0) normal (0, 0, 1) x (1, 0, 0)
  line L0 (30, 30) -> (-30, 30) construction
  line L1 (-30, 30) -> (-30, -30) construction
  line L2 (-30, -30) -> (30, -30) construction
  line L3 (30, -30) -> (30, 30) construction
  line L4 (30, 30) -> (-30, -30) construction
  line L5 (-30, 30) -> (30, -30) construction
  line L6 (-15.25, 15.25) -> (15.25, 15.25) construction
  line L7 (15.25, 15.25) -> (15.25, -15.25) construction
  line L8 (15.25, -15.25) -> (-15.25, -15.25) construction
  line L9 (-15.25, -15.25) -> (-15.25, 15.25) construction
  line L10 (-15.25, 15.25) -> (15.25, -15.25) construction
  line L11 (15.25, 15.25) -> (-15.25, -15.25) construction
  circle A0 centre (-15.25, 15.25) radius 2
  circle A1 centre (15.25, 15.25) radius 2
  circle A2 centre (-15.25, -15.25) radius 2
  circle A3 centre (15.25, -15.25) radius 2
  circle A4 centre (-30, 30) radius 1.6
  circle A5 centre (30, 30) radius 1.6
  circle A6 centre (30, -30) radius 1.6
  circle A7 centre (-30, -30) radius 1.6
  circle A8 centre (-30, 30) radius 8.1
  circle A9 centre (30, 30) radius 8.1
  circle A10 centre (30, -30) radius 8.1
  circle A11 centre (-30, -30) radius 8.1
  line L12 (0, 0) -> (19.7, 0) construction
  line L13 (35.7276, 24.2724) -> (25.8281, 14.3729)
  line L14 (35.7276, 24.2724) -> (49.642, 24.2724) construction
  line L15 (35.7276, -24.2724) -> (25.8281, -14.3729)
  line L16 (35.7276, -24.2724) -> (49.7976, -24.2724) construction
  arc A12 (25.8281, 14.3729) -> (25.8281, -14.3729) centre (39.6194, 0) ccw
  line L17 (0, 2.5) -> (0, 20)
  line L18 (-35.7276, -24.2724) -> (-25.8281, -14.3729)
  arc A13 (-25.8281, -14.3729) -> (-25.8281, 14.3729) centre (-39.6194, 0) ccw
  line L19 (-35.7276, 24.2724) -> (-25.8281, 14.3729)
  line L20 (0, 0) -> (0, -11.55) construction
  arc A14 (13, -20) -> (-13, -20) centre (0, -25.775) ccw
  spline S0 degree 5 poles (-13, -20) (-13.0721, -20.1624) (-13.2204, -20.4811) (-13.4544, -20.9411) (-13.7877, -21.5205) (-14.2264, -22.2015) (-14.6719, -22.8553) (-15.1114, -23.4963) (-15.5392, -24.1331) (-15.9624, -24.7634) (-16.3951, -25.379) (-16.8535, -25.9701) (-17.3506, -26.5301) (-17.8903, -27.0606) (-18.4641, -27.5747) (-19.0559, -28.0918) (-19.6462, -28.6332) (-20.2162, -29.2185) (-20.7523, -29.8604) (-21.2484, -30.5629) (-21.7028, -31.3245) (-22.0341, -31.9777) (-22.2655, -32.4902) (-22.4124, -32.8417) (-22.484, -33.0198) knots 0 0 0 0 0 0 0.05 0.1 0.15 0.2 0.25 0.3 0.35 0.4 0.45 0.5 0.55 0.6 0.65 0.7 0.75 0.8 0.85 0.9 0.95 1 1 1 1 1 1
  spline S1 degree 5 poles (13, -20) (13.0721, -20.1624) (13.2204, -20.4811) (13.4544, -20.9411) (13.7877, -21.5205) (14.2264, -22.2015) (14.6719, -22.8553) (15.1114, -23.4963) (15.5392, -24.1331) (15.9624, -24.7634) (16.3951, -25.379) (16.8535, -25.9701) (17.3506, -26.5301) (17.8903, -27.0606) (18.4641, -27.5747) (19.0559, -28.0918) (19.6462, -28.6332) (20.2162, -29.2185) (20.7523, -29.8604) (21.2484, -30.5629) (21.7028, -31.3245) (22.0341, -31.9777) (22.2655, -32.4902) (22.4124, -32.8417) (22.484, -33.0198) knots 0 0 0 0 0 0 0.05 0.1 0.15 0.2 0.25 0.3 0.35 0.4 0.45 0.5 0.55 0.6 0.65 0.7 0.75 0.8 0.85 0.9 0.95 1 1 1 1 1 1
  line L21 (-12.2466, -18.304) -> (-13.7534, -21.696)
  line L22 (-21.7921, -31.2978) -> (-23.1759, -34.7419)
  line L23 (12.2466, -18.304) -> (13.7534, -21.696)
  line L24 (21.7921, -31.2978) -> (23.1759, -34.7419)
  arc A15 (-13, 20) -> (13, 20) centre (0, 25.775) ccw
  spline S2 degree 5 poles (-13, 20) (-13.0721, 20.1624) (-13.2204, 20.4811) (-13.4544, 20.9411) (-13.7877, 21.5205) (-14.2264, 22.2015) (-14.6719, 22.8553) (-15.1114, 23.4963) (-15.5392, 24.1331) (-15.9624, 24.7634) (-16.3951, 25.379) (-16.8535, 25.9701) (-17.3506, 26.5301) (-17.8903, 27.0606) (-18.4641, 27.5747) (-19.0559, 28.0918) (-19.6462, 28.6332) (-20.2162, 29.2185) (-20.7523, 29.8604) (-21.2484, 30.5629) (-21.7028, 31.3245) (-22.0341, 31.9777) (-22.2655, 32.4902) (-22.4124, 32.8417) (-22.484, 33.0198) knots 0 0 0 0 0 0 0.05 0.1 0.15 0.2 0.25 0.3 0.35 0.4 0.45 0.5 0.55 0.6 0.65 0.7 0.75 0.8 0.85 0.9 0.95 1 1 1 1 1 1
  line L25 (-12.2466, 18.304) -> (-13.7534, 21.696)
  line L26 (-21.7921, 31.2978) -> (-23.1759, 34.7419)
  spline S3 degree 5 poles (13, 20) (13.0721, 20.1624) (13.2204, 20.4811) (13.4544, 20.9411) (13.7877, 21.5205) (14.2264, 22.2015) (14.6719, 22.8553) (15.1114, 23.4963) (15.5392, 24.1331) (15.9624, 24.7634) (16.3951, 25.379) (16.8535, 25.9701) (17.3506, 26.5301) (17.8903, 27.0606) (18.4641, 27.5747) (19.0559, 28.0918) (19.6462, 28.6332) (20.2162, 29.2185) (20.7523, 29.8604) (21.2484, 30.5629) (21.7028, 31.3245) (22.0341, 31.9777) (22.2655, 32.4902) (22.4124, 32.8417) (22.484, 33.0198) knots 0 0 0 0 0 0 0.05 0.1 0.15 0.2 0.25 0.3 0.35 0.4 0.45 0.5 0.55 0.6 0.65 0.7 0.75 0.8 0.85 0.9 0.95 1 1 1 1 1 1
  line L27 (12.2466, 18.304) -> (13.7534, 21.696)
  line L28 (21.7921, 31.2978) -> (23.1759, 34.7419)
  line L29 (0, -11.55) -> (0, -25.775) construction
  point P0 (-15.1252, -23.5197)
  point P1 (-17.2488, -26.4028)
  point P2 (-20.015, -29.0234)
  point P3 (15.1252, -23.5197)
  point P4 (17.2488, -26.4028)
  point P5 (20.015, -29.0234)
  point P6 (-15.1252, 23.5197)
  point P7 (-17.2488, 26.4028)
  point P8 (-20.015, 29.0234)
  point P9 (15.1252, 23.5197)
  point P10 (17.2488, 26.4028)
  point P11 (20.015, 29.0234)
  point P12 (0, -11.55)
  dimension "d1" = 60
  dimension "d2" = 60
  dimension "d3" = 30.5
  dimension "d4" = 30.5
  dimension "d5" = 4
  dimension "d7" = 3.2
  dimension "d8" = 16.2
  dimension "d9" = 19.7
  dimension "d10" = 135
  dimension "d11" = 14
  dimension "d12" = 135
  dimension "d13" = 14
  dimension "d14" = 11.55
  dimension "d15" = 20
  dimension "d16" = 13
  dimension "d17" = 13
  dimension "d18" = 20
  constraint horizontal L0
  constraint perpendicular L0 L1
  constraint parallel L0 L2
  constraint parallel L1 L3
  constraint coincident L4 L12.start
  constraint coincident L5 L12.start
  constraint coincident L12.start L20.start
  constraint horizontal L6
  constraint perpendicular L6 L7
  constraint parallel L6 L8
  constraint parallel L7 L9
  constraint coincident L10 L12.start
  constraint coincident L11 L12.start
  constraint coincident L6.start L9.end
  constraint coincident L6.end L7.start
  constraint coincident L8.end L9.start
  constraint coincident L7.end L8.start
  constraint equal A2 A3
  constraint equal A1 A2
  constraint equal A0 A1
  constraint coincident L0.end L1.start
  constraint coincident L0.start L3.end
  constraint coincident L2.end L3.start
  constraint coincident L1.end L2.start
  constraint equal A5 A6
  constraint equal A6 A7
  constraint equal A4 A7
  constraint concentric A4 A8
  constraint concentric A5 A9
  constraint concentric A6 A10
  constraint concentric A7 A11
  constraint equal A10 A11
  constraint equal A9 A10
  constraint equal A8 A9
  constraint horizontal L12
  constraint horizontal L14
  constraint coincident A9 L13.start
  constraint tangent A9 L13
  constraint horizontal L16
  constraint coincident A10 L15.start
  constraint tangent A10 L15
  constraint coincident L12.end A12
  constraint symmetric L13.start L17 L19.start
  constraint symmetric L13.end L17 A13.end
  constraint symmetric L15.start L17 L18.start
  constraint symmetric L15.end L17 L18.end
  constraint symmetric A12 L17 A13
  constraint vertical L20
  constraint coincident P12 A14
  constraint coincident A11 S0.end
  constraint tangent A14 S0
  constraint tangent A11 S0
  constraint midpoint A14.end L21
  constraint midpoint S0.end L22
  constraint symmetric L20 A14.end A14.start
  constraint symmetric L20 P0 P3
  constraint symmetric L20 P1 P4
  constraint symmetric L20 P2 P5
  constraint symmetric L20 S0.end S1.end
  constraint symmetric L20 L21.start L23.start
  constraint symmetric L20 L21.end L23.end
  constraint symmetric L20 L22.start L24.start
  constraint symmetric L20 L22.end L24.end
  constraint symmetric L12 A14.end A15.start
  constraint symmetric L12 A14.start A15.end
  constraint symmetric L12 A14 A15
  constraint symmetric L12 P0 P6
  constraint symmetric L12 P1 P7
  constraint symmetric L12 P2 P8
  constraint symmetric L12 S0.end S2.end
  constraint symmetric L12 P3 P9
  constraint symmetric L12 P4 P10
  constraint symmetric L12 P5 P11
  constraint symmetric L12 S1.end S3.end
  constraint symmetric L12 L21.start L25.start
  constraint symmetric L12 L21.end L25.end
  constraint symmetric L12 L22.start L26.start
  constraint symmetric L12 L22.end L26.end
  constraint symmetric L12 L23.start L27.start
  constraint symmetric L12 L23.end L27.end
  constraint symmetric L12 L24.start L28.start
  constraint symmetric L12 L24.end L28.end
  constraint coincident P12 L20.end
  constraint coincident A14.centre L29.end
  measures "d1" distance of L1.end L2.end
  measures "d2" distance of L0.end L1.end
  measures "d3" distance of L7.end L8.end
  measures "d4" distance of L6.end L7.end
  measures "d5" diameter of A0
  measures "d7" diameter of A4
  measures "d8" diameter of A8
  measures "d9" distance of L12.start L12.end
  measures "d10" angle of L13 L14
  measures "d11" distance of L13.start L13.end
  measures "d12" angle of L15 L16
  measures "d13" distance of L15.start L15.end
  measures "d14" distance of L12.start P12
  measures "d15" vertical distance of L12.start A14.start
  measures "d16" horizontal distance of L12.start A14.start
  measures "d17" horizontal distance of L12.start A14.end
  measures "d18" vertical distance of L12.start A14.end
extrude "Extrude1" add sketch "Sketch1" along normal blind 2
equation "d9 = ( 39.4 / 2 ) * 1 mm"
equation "d14 = ( 23.1 / 2 ) * 1 mm"
equation "d17 = d16"
equation "d18 = d15"

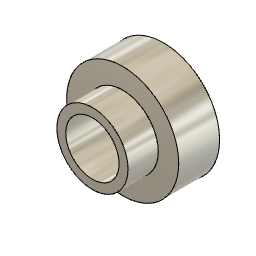
design "press_nut"
Autodesk Fusion 360 part; units mm, degrees
sketch "Sketch1" plane through (0, 0, 0) normal (0, 0, 1) x (1, 0, 0)
  circle A0 centre (0, 0) radius 3.15
  circle A1 centre (0, 0) radius 1.5
  dimension "d1" = 6.3
  dimension "d2" = 3
  constraint coincident A0.centre A1.centre
  measures "d1" diameter of A0
  measures "d2" diameter of A1
extrude "Extrude1" add sketch "Sketch1" along normal blind 4
sketch "Sketch2" plane through (0, 0, 4) normal (0, 0, 1) x (1, 0, 0)
  circle A0 centre (0, 0) radius 1.5
  circle A1 centre (0, 0) radius 3.15
  circle A2 centre (0, 0) radius 2
  dimension "d5" = 4
  constraint concentric A0 A2
  measures "d5" diameter of A2
extrude "Extrude2" cut sketch "Sketch2" against normal blind 1.7 contours A1

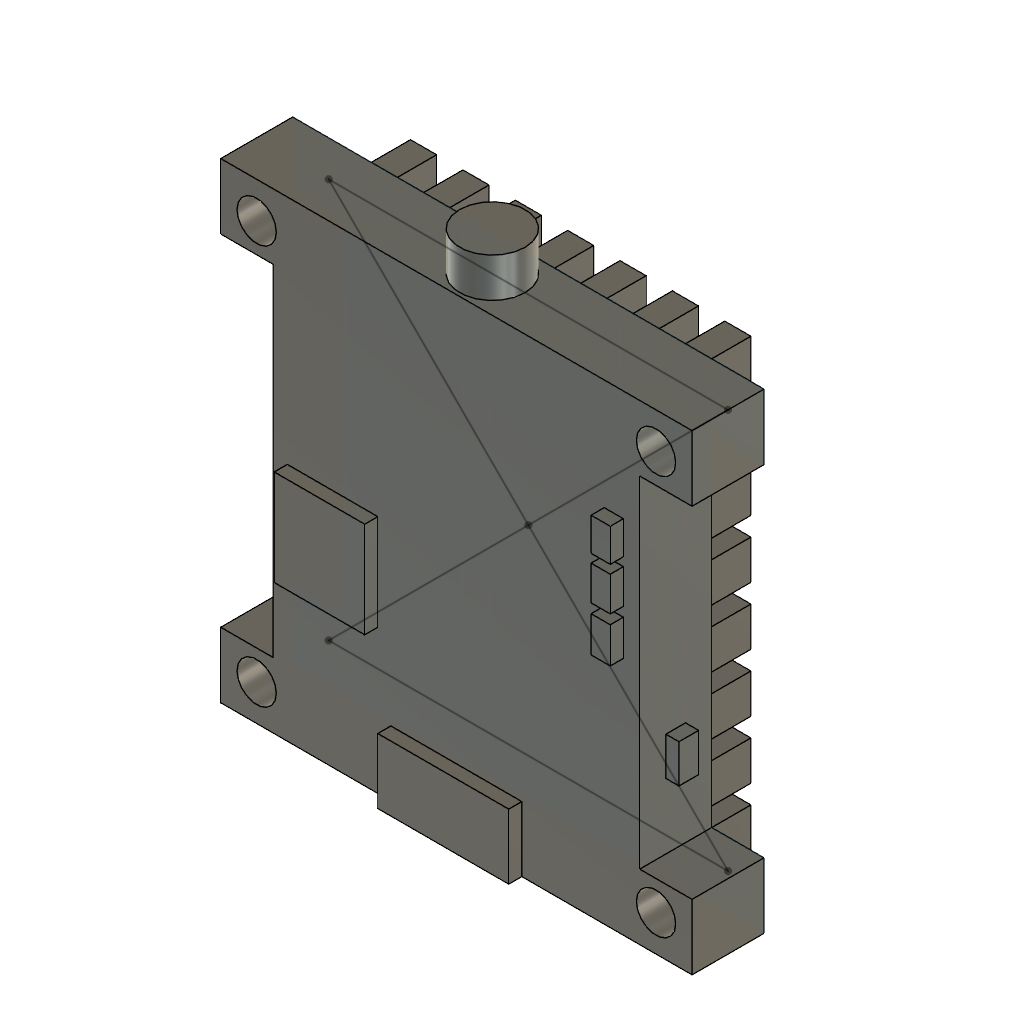
design "vtx_model"
part number: 2026-09-24-17-20-19-452
Autodesk Fusion 360 part; units mm, degrees
sketch "Sketch1" plane through (0, 0, 0) normal (0, 1, 0) x (1, 0, 0)
  line L0 (0, 0) -> (36, 0)
  line L1 (36, 0) -> (36, -36)
  line L2 (36, -36) -> (0, -36)
  line L3 (0, -36) -> (0, 0)
  dimension "d1" = 36
  dimension "d2" = 36
  constraint horizontal L0
  constraint vertical L1
  constraint horizontal L2
  constraint vertical L3
  constraint coincident L0.start L3.end
  measures "d1" distance of L0.start L0.end
  measures "d2" distance of L0.end L1.end
extrude "Extrude1" add sketch "Sketch1" along normal blind 5.5
form "Form1" [no effect]
sketch "Sketch2" plane through (0, 0, 0) normal (0, -1, 0) x (1, 0, 0)
  line L0 (36, 36) -> (0, 36)
  line L1 (0, 36) -> (0, 0)
  line L2 (0, 0) -> (36, 0)
  line L3 (36, 0) -> (36, 36)
  line L4 (2.75, 33.25) -> (33.25, 33.25)
  line L5 (33.25, 33.25) -> (33.25, 2.75)
  line L6 (33.25, 2.75) -> (2.75, 2.75)
  line L7 (2.75, 2.75) -> (2.75, 33.25)
  circle A0 centre (33.25, 33.25) radius 1.5
  circle A1 centre (2.75, 33.25) radius 1.5
  circle A2 centre (33.25, 2.75) radius 1.5
  circle A3 centre (2.75, 2.75) radius 1.5
  dimension "d12" = 3
  dimension "d13" = 3
  dimension "d14" = 3
  dimension "d15" = 3
  constraint horizontal L4
  constraint vertical L5
  constraint horizontal L6
  constraint vertical L7
  constraint coincident L4.end L5.start
  constraint coincident L4.start L7.end
  constraint coincident L5.end L6.start
  constraint coincident L6.end L7.start
  measures "d12" diameter of A0
  measures "d13" diameter of A1
  measures "d14" diameter of A2
  measures "d15" diameter of A3
extrude "Extrude2" cut sketch "Sketch2" against normal blind 15 contours L4 L7 A1 | L4 L7 A1 | L4 L5 A0 | L4 L5 A0 | L6 L7 A3 | L6 L7 A3 | L5 L6 A2 | L5 L6 A2
sketch "Sketch3" plane through (0, 5.5, 0) normal (0, 1, 0) x (-1, 0, 0)
  circle A0 centre (-2.75, 33.25) radius 1.5
  circle A1 centre (-2.75, 2.75) radius 1.5
  circle A2 centre (-33.25, 33.25) radius 1.5
  circle A3 centre (-33.25, 2.75) radius 1.5
  line L0 (0, 36) -> (-36, 36)
  line L1 (-36, 36) -> (-36, 0)
  line L2 (-36, 0) -> (0, 0)
  line L3 (0, 0) -> (0, 36)
  line L4 (-34.3236, 34.2975) -> (-1.8525, 34.2975)
  line L5 (-1.8525, 34.2975) -> (-1.8525, 1.5482)
  line L6 (-1.8525, 1.5482) -> (-34.3236, 1.5482)
  line L7 (-34.3236, 1.5482) -> (-34.3236, 34.2975)
  constraint horizontal L4
  constraint vertical L5
  constraint horizontal L6
  constraint vertical L7
  constraint coincident A1 L5.end
  constraint coincident A2 L4.start
sketch "Sketch4" plane through (0, 5.5, 0) normal (0, 1, 0) x (-1, 0, 0)
  circle A0 centre (-2.75, 33.25) radius 1.5
  circle A1 centre (-2.75, 2.75) radius 1.5
  circle A2 centre (-33.25, 33.25) radius 1.5
  circle A3 centre (-33.25, 2.75) radius 1.5
  line L0 (0, 36) -> (-36, 36)
  line L1 (-36, 36) -> (-36, 0)
  line L2 (-36, 0) -> (0, 0)
  line L3 (0, 0) -> (0, 36)
  line L4 (-31, 35) -> (-29, 35)
  line L5 (-29, 35) -> (-29, 32)
  line L6 (-29, 32) -> (-31, 32)
  line L7 (-31, 32) -> (-31, 35)
  dimension "d20" = 3
  constraint horizontal L4
  constraint vertical L5
  constraint horizontal L6
  constraint vertical L7
  measures "d20" distance of L4.start L6.end
extrude "Extrude4" add sketch "Sketch4" along normal blind 4 contours L4 L5 L6 L7
pattern_linear "R-Pattern1" count 8 spacing 4.4286 along (0, 0, -1) count 7 spacing 4 along (-1, 0, 0) of "Extrude4"